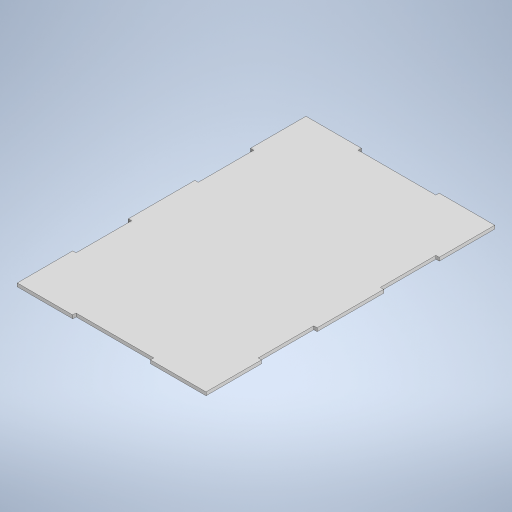
# Autodesk Inventor part: Alas Bawah
Saved by Autodesk Inventor 2024 (Build 280153000, 153)
## iProperties
Created: 2023-07-10
Part Number: Alas Bawah
Material: Generic
Document SubType Name: Modeling
Designer: Asus
Density: 1 g/cm^3
Appearance: Default
Author: Asus
Autodesk Inventor part; units mm, degrees
ref_plane "YZ Plane" through (0, 0, 0) normal (1, 0, 0) x (0, 1, 0)
ref_plane "XZ Plane" through (0, 0, 0) normal (0, 1, 0) x (-1, 0, 0)
ref_plane "XY Plane" through (0, 0, 0) normal (0, 0, 1) x (1, 0, 0)
sketch "Sketch2" plane through (0, 0, 0) normal (0, 1, 0) x (-1, 0, 0)
  line L0 (0, 0) -> (0, -50)
  line L1 (0, -50) -> (3, -50)
  line L2 (3, -50) -> (3, -100)
  line L3 (3, -100) -> (0, -100)
  line L4 (0, -100) -> (0, -160)
  line L5 (0, -160) -> (3, -160)
  line L6 (3, -160) -> (3, -210)
  line L7 (3, -210) -> (0, -210)
  line L8 (0, -210) -> (0, -260)
  line L9 (0, -260) -> (50, -260)
  line L10 (50, -260) -> (50, -257)
  line L11 (50, -257) -> (120, -257)
  line L12 (120, -257) -> (120, -260)
  line L13 (120, -260) -> (170, -260)
  line L14 (170, 0) -> (120, 0)
  line L15 (120, 0) -> (120, -3)
  line L16 (120, -3) -> (50, -3)
  line L17 (50, -3) -> (50, 0)
  line L18 (50, 0) -> (0, 0)
  line L19 (170, 0) -> (170, -50)
  line L20 (170, -50) -> (167, -50)
  line L21 (167, -50) -> (167, -100)
  line L22 (167, -100) -> (170, -100)
  line L23 (170, -100) -> (170, -160)
  line L24 (170, -160) -> (167, -160)
  line L25 (167, -160) -> (167, -210)
  line L26 (167, -210) -> (170, -210)
  line L27 (170, -210) -> (170, -260)
  dimension "d2" = 50
  dimension "d3" = 3
  dimension "d4" = 50
  dimension "d5" = 3
  dimension "d6" = 60
  dimension "d7" = 50
  dimension "d8" = 50
  dimension "d9" = 50
  dimension "d10" = 3
  dimension "d11" = 70
  dimension "d12" = 50
  dimension "d18" = 50
  dimension "d19" = 3
  dimension "d20" = 70
  dimension "d23" = 50
  dimension "d28" = 50
  dimension "d29" = 3
  dimension "d30" = 50
  dimension "d31" = 3
  dimension "d32" = 60
  dimension "d36" = 3
  dimension "d37" = 50
  dimension "d38" = 3
  constraints: 56 end point, 17 perpendicular, 11 point on line, 2 vertical, 1 horizontal
  measures "d2" distance of L0.start L0.end
  measures "d3" distance of L0.end L1.end
  measures "d4" distance of L1.end L2.end
  measures "d5" distance of L2.end L3.end
  measures "d6" distance of L3.end L4.end
  measures "d7" distance of L5.end L6.end
  measures "d8" distance of L7.end L8.end
  measures "d9" distance of L8.end L9.end
  measures "d10" distance of L9.end L10.end
  measures "d11" distance of L10.end L11.end
  measures "d12" distance of L12.end L13.end
  measures "d18" distance of L14.start L14.end
  measures "d19" distance of L14.end L15.end
  measures "d20" distance of L15.end L16.end
  measures "d23" distance of L17.end L0.start
  measures "d28" distance of L14.start L19.end
  measures "d29" distance of L19.end L20.end
  measures "d30" distance of L20.end L21.end
  measures "d31" distance of L21.end L22.end
  measures "d32" distance of L22.end L23.end
  measures "d36" distance of L23.end L24.end
  measures "d37" distance of L24.end L25.end
  measures "d38" distance of L25.end L26.end
extrude "Extrusion1" add sketch "Sketch2" along normal blind 3
body "Solid1"
